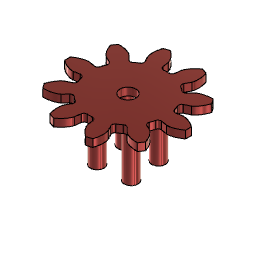
Gear Middle with Tubes (Autodesk Fusion 360 design; units mm, degrees)
description: Spur Gear; Module: 10.0; Num Teeth: 10; Pressure Angle: 20.0; Backlash: 0.00 mm
Autodesk Fusion 360 part; units mm, degrees
note: some values were not read from the file. Set by a fixed rule: which face or edge a step refers to.
sketch "Base" plane through (0, 0, 0) normal (0, 0, 1) x (1, 0, 0)
  circle A0 centre (0, 0) radius 37.9492
  circle A1 centre (0, 0) radius 1.5
extrude "Extrude1" add sketch "Base" along normal blind 3
sketch "Tooth" plane through (0, 0, 0) normal (0, 0, 1) x (1, 0, 0)
  spline S0 degree 5 poles (46.2915, -8.0408) (46.3305, -8.0476) (46.4086, -8.0598) (46.5261, -8.0739) (46.6835, -8.0849) (46.8813, -8.0882) (47.0798, -8.084) (47.2787, -8.0754) (47.4778, -8.0643) (47.677, -8.0515) (47.8764, -8.0367) (48.0758, -8.0194) (48.2754, -7.9987) (48.4751, -7.9742) (48.675, -7.9459) (48.8749, -7.9143) (49.0749, -7.8797) (49.2749, -7.8428) (49.4748, -7.8037) (49.6747, -7.7626) (49.8745, -7.7194) (50.0742, -7.6739) (50.2739, -7.626) (50.4734, -7.5758) (50.6729, -7.5232) (50.8722, -7.4684) (51.0714, -7.4115) (51.2705, -7.3526) (51.4694, -7.2918) (51.6681, -7.229) (51.8666, -7.1643) (52.0649, -7.0977) (52.2631, -7.0291) (52.461, -6.9587) (52.6587, -6.8864) (52.8562, -6.8122) (53.0534, -6.7362) (53.2504, -6.6585) (53.4471, -6.579) (53.6436, -6.4978) (53.8398, -6.4148) (54.0357, -6.3302) (54.2313, -6.2439) (54.4266, -6.1559) (54.6216, -6.0662) (54.8162, -5.9749) (55.0106, -5.8819) (55.2046, -5.7874) (55.3983, -5.6913) (55.5917, -5.5935) (55.7847, -5.4943) (55.9773, -5.3934) (56.1696, -5.2911) (56.3615, -5.1872) (56.553, -5.0818) (56.7441, -4.9748) (56.9349, -4.8664) (57.1252, -4.7565) (57.3151, -4.6452) (57.5046, -4.5324) (57.6937, -4.4181) (57.8824, -4.3024) (58.0707, -4.1853) (58.2585, -4.0668) (58.4459, -3.9468) (58.6328, -3.8255) (58.8193, -3.7027) (59.0053, -3.5786) (59.1908, -3.4532) (59.3758, -3.3263) (59.5604, -3.1981) (59.7077, -3.0945) (59.818, -3.0162) (59.8914, -2.9637) (59.9281, -2.9374) knots 0 0 0 0 0 0 0.01428571 0.02857143 0.04285714 0.05714286 0.07142857 0.08571429 0.1 0.11428571 0.12857143 0.14285714 0.15714286 0.17142857 0.18571429 0.2 0.21428571 0.22857143 0.24285714 0.25714286 0.27142857 0.28571429 0.3 0.31428571 0.32857143 0.34285714 0.35714286 0.37142857 0.38571429 0.4 0.41428571 0.42857143 0.44285714 0.45714286 0.47142857 0.48571429 0.5 0.51428571 0.52857143 0.54285714 0.55714286 0.57142857 0.58571429 0.6 0.61428571 0.62857143 0.64285714 0.65714286 0.67142857 0.68571429 0.7 0.71428571 0.72857143 0.74285714 0.75714286 0.77142857 0.78571429 0.8 0.81428571 0.82857143 0.84285714 0.85714286 0.87142857 0.88571429 0.9 0.91428571 0.92857143 0.94285714 0.95714286 0.97142857 0.98571429 1 1 1 1 1 1
  spline S1 degree 5 poles (46.2915, 8.0408) (46.3305, 8.0476) (46.4086, 8.0598) (46.5261, 8.0739) (46.6835, 8.0849) (46.8813, 8.0882) (47.0798, 8.084) (47.2787, 8.0754) (47.4778, 8.0643) (47.677, 8.0515) (47.8764, 8.0367) (48.0758, 8.0194) (48.2754, 7.9987) (48.4751, 7.9742) (48.675, 7.9459) (48.8749, 7.9143) (49.0749, 7.8797) (49.2749, 7.8428) (49.4748, 7.8037) (49.6747, 7.7626) (49.8745, 7.7194) (50.0742, 7.6739) (50.2739, 7.626) (50.4734, 7.5758) (50.6729, 7.5232) (50.8722, 7.4684) (51.0714, 7.4115) (51.2705, 7.3526) (51.4694, 7.2918) (51.6681, 7.229) (51.8666, 7.1643) (52.0649, 7.0977) (52.2631, 7.0291) (52.461, 6.9587) (52.6587, 6.8864) (52.8562, 6.8122) (53.0534, 6.7362) (53.2504, 6.6585) (53.4471, 6.579) (53.6436, 6.4978) (53.8398, 6.4148) (54.0357, 6.3302) (54.2313, 6.2439) (54.4266, 6.1559) (54.6216, 6.0662) (54.8162, 5.9749) (55.0106, 5.8819) (55.2046, 5.7874) (55.3983, 5.6913) (55.5917, 5.5935) (55.7847, 5.4943) (55.9773, 5.3934) (56.1696, 5.2911) (56.3615, 5.1872) (56.553, 5.0818) (56.7441, 4.9748) (56.9349, 4.8664) (57.1252, 4.7565) (57.3151, 4.6452) (57.5046, 4.5324) (57.6937, 4.4181) (57.8824, 4.3024) (58.0707, 4.1853) (58.2585, 4.0668) (58.4459, 3.9468) (58.6328, 3.8255) (58.8193, 3.7027) (59.0053, 3.5786) (59.1908, 3.4532) (59.3758, 3.3263) (59.5604, 3.1981) (59.7077, 3.0945) (59.818, 3.0162) (59.8914, 2.9637) (59.9281, 2.9374) knots 0 0 0 0 0 0 0.01428571 0.02857143 0.04285714 0.05714286 0.07142857 0.08571429 0.1 0.11428571 0.12857143 0.14285714 0.15714286 0.17142857 0.18571429 0.2 0.21428571 0.22857143 0.24285714 0.25714286 0.27142857 0.28571429 0.3 0.31428571 0.32857143 0.34285714 0.35714286 0.37142857 0.38571429 0.4 0.41428571 0.42857143 0.44285714 0.45714286 0.47142857 0.48571429 0.5 0.51428571 0.52857143 0.54285714 0.55714286 0.57142857 0.58571429 0.6 0.61428571 0.62857143 0.64285714 0.65714286 0.67142857 0.68571429 0.7 0.71428571 0.72857143 0.74285714 0.75714286 0.77142857 0.78571429 0.8 0.81428571 0.82857143 0.84285714 0.85714286 0.87142857 0.88571429 0.9 0.91428571 0.92857143 0.94285714 0.95714286 0.97142857 0.98571429 1 1 1 1 1 1
  arc A0 (59.9281, -2.9374) -> (59.9281, 2.9374) centre (0, 0) ccw
  line L0 (37.3795, -6.4945) -> (46.2915, -8.0408)
  line L1 (37.3795, 6.4945) -> (46.2915, 8.0408)
  line L2 (37.3795, -6.4945) -> (37.3795, 6.4945)
  point P0 (47.2286, -8.0771)
  point P1 (48.1831, -8.0078)
  point P2 (49.1482, -7.8659)
  point P3 (50.121, -7.6623)
  point P4 (51.0995, -7.4028)
  point P5 (52.0821, -7.0913)
  point P6 (53.0672, -6.7304)
  point P7 (54.0535, -6.3219)
  point P8 (55.0398, -5.8674)
  point P9 (56.0248, -5.3679)
  point P10 (57.0072, -4.8244)
  point P11 (57.986, -4.2378)
  point P12 (58.96, -3.6085)
  point P13 (47.2286, 8.0771)
  point P14 (48.1831, 8.0078)
  point P15 (49.1482, 7.8659)
  point P16 (50.121, 7.6623)
  point P17 (51.0995, 7.4028)
  point P18 (52.0821, 7.0913)
  point P19 (53.0672, 6.7304)
  point P20 (54.0535, 6.3219)
  point P21 (55.0398, 5.8674)
  point P22 (56.0248, 5.3679)
  point P23 (57.0072, 4.8244)
  point P24 (57.986, 4.2378)
  point P25 (58.96, 3.6085)
extrude "Extrude2" add sketch "Tooth" along normal blind 3
fillet "Fillet1" radius 3 2 edges at (37.3891, -6.4962, 1.5) (37.3891, 6.4962, 1.5)
pattern_circular "C-Pattern1" count 10 over 360 about axis through (0, 0, 0) along (0, 0, 1) of "Extrude2", "Fillet1"
scale "Scale1" factor 0.2 about (-1.5, 0, 3) bodies 1
scale "Scale2" factor 1.1 about (-1.5, 0, 3) bodies 1
move_face "OffsetFaces1" offset -0.7 1 faces at (-0.8404, -0.0164, 2.78)
extrude "Extrude3" add 1 faces at (0.6395, 5.5026, 2.34) along direction (0, 0, -1) blind 1
move_face "OffsetFaces2" offset -1 2 faces at (-0.1451, -0.1026, 2.0067) (-0.1413, -0.0513, 2.78)
move_face "OffsetFaces3" offset 0.3 1 faces at (0.8499, 0.2021, 2.4467)
sketch "Holes for Tubes" plane through (0, 0, 3) normal (0, 0, 1) x (-1, 0, 0)
  circle A0 centre (-2.5, 3) radius 1.5
  circle A1 centre (1.2, 0) radius 5.5172
  circle A2 centre (-1.8, -3.7) radius 1.5
  circle A3 centre (4.9, -3) radius 1.5
  circle A4 centre (4.2, 3.7) radius 1.5
  dimension "d284" = 3
  dimension "d286" = 360
  measures "d284" diameter of A0
extrude "Extrude4" cut sketch "Holes for Tubes" against normal blind 16 contours A0 A1 | A0 A1 | A1 A4 | A1 A4 | A1 A2 | A1 A2 | A1 A3 | A1 A3
extrude "Extrude5" add sketch "Holes for Tubes" against normal blind 13 contours A0 A1 | A0 A1 | A1 A4 | A1 A4 | A1 A2 | A1 A2 | A1 A3 | A1 A3
named bodies: "Base for Wheel with tubes"
